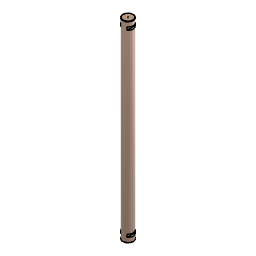
thermal conductor v6 (Autodesk Fusion 360 design; units mm, degrees)
Autodesk Fusion 360 part; units mm, degrees
sketch "Sketch1" plane through (0, 0, 0) normal (0, 0, 1) x (1, 0, 0)
  line L0 (-7.5, 0) -> (7.5, 0)
  line L1 (7.5, 0) -> (7.5, 275)
  line L2 (7.5, 275) -> (-7.5, 275)
  line L3 (-7.5, 275) -> (-7.5, 0)
  line L4 (-7.5, 7) -> (-4.5, 7)
  line L5 (-4.5, 7) -> (-4.5, 11)
  line L6 (-4.5, 11) -> (-7.5, 11)
  line L7 (0, 0) -> (0, 275)
  dimension "d1" = 15
  dimension "d2" = 275
  dimension "d3" = 7
  dimension "d4" = 4
  dimension "d5" = 3
  constraint horizontal L0
  constraint perpendicular L0 L1
  constraint perpendicular L1 L2
  constraint perpendicular L0 L3
  constraint midpoint L7.start L0
  constraint coincident L3 L4.start
  constraint perpendicular L3 L4
  constraint perpendicular L4 L5
  constraint coincident L3 L6.end
  constraint perpendicular L3 L6
  constraint coincident L7.start origin
  constraint midpoint L2 L7.end
  measures "d1" distance of L1 L3
  measures "d2" distance of L0.end L1.end
  measures "d3" distance of L0 L4
  measures "d4" distance of L4.end L5.end
  measures "d5" distance of L3 L5
revolve "Revolve1" add sketch "Sketch1" angle 360 about axis through (0, 0, 0) along (0, 1, 0) contours L0 L1 L2 L7
extrude "Extrude1" cut sketch "Sketch1" along normal through all and the other way through all contours L3 L4 L5 L6
mirror "Mirror1" about plane through (0, 0, 0) normal (1, 0, 0) of "Extrude1"
ref_plane "WorkPlane1" through (0, 137.5, 0) normal (0, -1, 0) x (0, 0, -1)
hole "Hole2" at (0, 0, 0) direction (0, 1, 0) diameter 1.5 depth 5 tip angle 118
mirror "Mirror2" about plane through (0, 137.5, 0) normal (0, -1, 0) of "Extrude1", "Mirror1", "Hole2"
chamfer "Chamfer1" distance 0.5 angle 45 2 edges at (-6.9925, 0, -2.7121) (-6.9925, 275, -2.7121)
